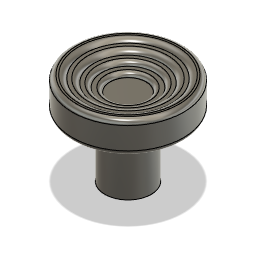
Warthog Slew Stick v11 (Autodesk Fusion 360 design; units mm, degrees)
Autodesk Fusion 360 part; units mm, degrees
note: some values were not read from the file. Set by a fixed rule: which face or edge a step refers to.
sketch "Sketch1" plane through (0, 0, 0) normal (0, 1, 0) x (1, 0, 0)
  circle A0 centre (0, 0) radius 6
  circle A1 centre (0, 0) radius 5
  circle A2 centre (0, 0) radius 4
  circle A3 centre (0, 0) radius 3
  constraint coincident A0.centre A1.centre
  constraint concentric A0 A1
  constraint concentric A0 A2
  constraint concentric A1 A3
extrude "Extrude1" add sketch "Sketch1" along normal blind 5 contours A0 makes body 1
sketch "Sketch2" plane through (0, 0, 0) normal (0, 1, 0) x (1, 0, 0)
  circle A0 centre (0, 0) radius 5
  circle A1 centre (0, 0) radius 4
  constraint coincident A0.centre A1.centre
  constraint concentric A0 A1
extrude "Extrude2" add sketch "Sketch2" along normal blind 4 bodies 1
sketch "Sketch3" plane through (0, 0, 0) normal (0, 1, 0) x (1, 0, 0)
  circle A0 centre (0, 0) radius 4
  circle A1 centre (0, 0) radius 3
  constraint coincident A0.centre A1.centre
extrude "Extrude3" add sketch "Sketch3" along normal blind 3 bodies 1
sketch "Sketch4" plane through (0, 0, 0) normal (0, 1, 0) x (1, 0, 0)
  circle A0 centre (0, 0) radius 3
  constraint coincident A0.centre origin
extrude "Extrude4" add sketch "Sketch4" along normal blind 2 bodies 1
sketch "Sketch5" plane through (0, 2, 0) normal (0, 1, 0) x (-1, 0, 0)
  circle A0 centre (0, 0) radius 3
extrude "Extrude5" add 1 faces at (4.6332, 4, 0.4471) along direction (0, 1, 0) blind 0.5 on bodies 1 bodies 1
extrude "Extrude6" add 1 faces at (3.6406, 3, 0.3478) along direction (0, 1, 0) blind 1 on bodies 1 bodies 1
extrude "Extrude7" add sketch "Sketch5" along normal blind 1.5 bodies 1
extrude "Extrude8" cut 1 faces at (-1.0665, 0, -0.3664) along direction (0, 1, 0) blind 1 on bodies 1 bodies 1
extrude "Extrude9" cut 1 faces at (-1.0665, 1, -0.3664) along direction (0, 1, 0) blind 0.5 on bodies 1 bodies 1
sketch "Sketch6" plane through (0, 0, 0) normal (0, 1, 0) x (1, 0, 0)
  circle A0 centre (16.439, 2.6378) radius 2.4998
  line L0 (15.1107, 1.1426) -> (17.7673, 1.1426)
  line L1 (15.1107, 4.133) -> (17.7673, 4.133)
  circle A1 centre (16.439, 2.6378) radius 2
  constraint concentric A0 A1
  constraint coincident L1.start A1
  constraint coincident L1.end A1
  constraint horizontal L1
  constraint coincident L0.start A1
  constraint coincident L0.end A1
  constraint parallel L0 L1
extrude "Extrude10" add sketch "Sketch6" along normal blind 6 separate body contours A0 | L0 A1 | L1 A1 makes body 2
fillet "Fillet1" radius 0.5 1 edges at (-5.594, 5, 2.1697) on bodies 1
move_body "Align1" bodies 1 to x (1, 0, 0) y (0, 1, 0) z (0, 0, 1) at (16.439, 4.5, -2.6378)
extrude "Extrude11" add 1 faces at (21.0722, 9, -2.1907) along direction (0, 1, 0) blind 0.25 on bodies 1 bodies 1
extrude "Extrude12" add 1 faces at (20.0796, 8.5, -2.29) along direction (0, 1, 0) blind 0.5 on bodies 1 bodies 1
extrude "Extrude13" add 1 faces at (17.285, 8, -2.4447) along direction (0, 1, 0) blind 0.75 on bodies 1 bodies 1
extrude "Extrude14" cut 1 faces at (15.3725, 6, -3.0041) along direction (0, 1, 0) blind 1 on bodies 1 bodies 1
move_body "Move1" bodies 1 to x (1, 0, 0) y (0, 1, 0) z (0, 0, 1) at (0, -1, 0)
fillet "Fillet2" radius 0.3 1 edges at (13.642, 8, -3.7226) on bodies 1
fillet "Fillet3" radius 0.3 1 edges at (12.7097, 8.25, -4.0842) on bodies 1
fillet "Fillet4" radius 0.3 1 edges at (11.7774, 8.5, -4.4459) on bodies 1
extrude "Extrude15" add 1 faces at (16.3767, 0, -4.4655) along direction (0, -1, 0) blind 1 on bodies 2 bodies 2
fillet "Fillet5" radius 0.5 1 edges at (10.8451, 6, -0.4681) on bodies 1
combine "Combine1" operation add target body 1 tool bodies 2
scale "Scale1" factor 1.17647 about (15.1107, 6, -1.1426) bodies 1
scale "Scale2" factor 0.97 about (10.2028, 6, -2.9016) bodies 1
move_face "OffsetFaces1" offset -1 1 faces at (16.9098, 6, -2.4094) on bodies 1
chamfer "Chamfer1" distance 1.7 angle 45 1 faces at (17.0594, 7, -2.4094) on bodies 1
move_face "OffsetFaces2" offset 0.5 1 faces at (21.5805, 6, -2.4481) on bodies 1
move_face "OffsetFaces3" offset 0.5 1 faces at (21.4073, 8.8529, 0.8356) on bodies 1
move_face "OffsetFaces4" offset 0.4 1 faces at (21.5492, 8.5676, -3.4042) on bodies 1
move_face "OffsetFaces5" offset 0.2 1 faces at (20.497, 8.2824, -3.1087) on bodies 1
sketch "Sketch7" plane through (0, 7.9971, 0) normal (0, 1, 0) x (-1, 0, 0)
  circle A0 centre (-16.4793, -2.9016) radius 3.2217
  circle A1 centre (-16.4793, -2.9016) radius 2.2182
  constraint concentric A0 A1
extrude "Extrude16" cut sketch "Sketch7" against normal blind 0.5 contours A1 bodies 1
fillet "Fillet6" radius 0.5 1 edges at (18.5474, 7.9971, -2.0995) on bodies 1
scale "Scale3" factor 0.954 about (22.5228, 9.3529, -2.9016) bodies 1
